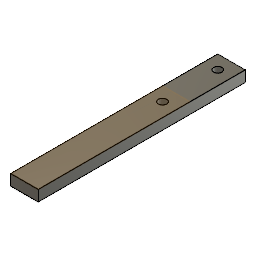
Endstop Pusher (Autodesk Fusion 360 design; units mm, degrees)
Autodesk Fusion 360 part; units mm, degrees
sketch "Skizze1" plane through (0, 0, 0) normal (0, 1, 0) x (1, 0, 0)
  line L0 (0, 0) -> (10, 0)
  line L1 (10, 0) -> (10, -40)
  line L2 (0, 0) -> (0, -40)
  line L3 (10, -40) -> (10, -45)
  line L4 (0, -40) -> (0, -45)
  line L5 (0, -45) -> (10, -45)
  constraint coincident L0.start L2.start
  constraint horizontal L0
  constraint perpendicular L0 L1
  constraint vertical L2
  constraint parallel L1 L3
  constraint parallel L2 L4
  constraint perpendicular L3 L5
extrude "Extrusion1" add sketch "Skizze1" along normal blind 4
sketch "Skizze2" plane through (0, 4, 0) normal (0, 1, 0) x (-1, 0, 0)
  line L0 (0, 0) -> (0, 45)
  line L1 (0, 45) -> (-10, 45)
  line L2 (-10, 45) -> (-10, 0)
  line L3 (-10, 0) -> (0, 0)
  circle A0 centre (-5, 5) radius 1.5
  dimension "d3" = 3
  measures "d3" diameter of A0
extrude "Extrusion2" cut sketch "Skizze2" against normal blind 24 contours A0
extrude "Extrusion3" add 1 faces at (3.3333, 1.3333, 45) along direction (0, 0, 1) blind 10
sketch "Skizze3" plane through (0, 4, 0) normal (0, 1, 0) x (-1, 0, 0)
  circle A0 centre (-5, 5) radius 1.5
  line L0 (0, 0) -> (0, 55)
  line L1 (0, 55) -> (-10, 55)
  line L2 (-10, 55) -> (-10, 0)
  line L3 (-10, 0) -> (0, 0)
extrude "Extrusion4" add 1 faces at (3.3333, 1.3333, 0) along direction (0, 0, -1) blind 20
sketch "Skizze4" plane through (0, 4, 0) normal (0, 1, 0) x (-1, 0, 0)
  circle A0 centre (-5, 5) radius 1.5
  line L0 (0, -20) -> (0, 55)
  line L1 (0, 55) -> (-10, 55)
  line L2 (-10, 55) -> (-10, -20)
  line L3 (-10, -20) -> (0, -20)
  circle A1 centre (-5, -15) radius 1.5
  dimension "d10" = 3
  measures "d10" diameter of A1
extrude "Extrusion5" cut sketch "Skizze4" against normal blind 15 contours A1
